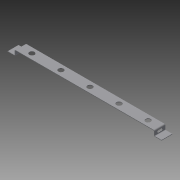
# Autodesk Inventor part: LEDStripOrigami
Saved by Autodesk Inventor 2016 (Build 200138000, 138)
## iProperties
Created: 2015-05-11
Part Number: LEDStripOrigami
Material: Generic
Document SubType Name: Sheet Metal
Designer: Erin
Density: 1 g/cm^3
Sheet Metal Rule: Default_mm
Appearance: Default
Flat Pattern Width: 1 cm
Flat Pattern Length: 15.0524 cm
Flat Pattern Area: 15.0524 cm^2
Sheet Metal Width: 10.000 mm
Sheet Metal Length: 150.524 mm
Sheet Metal Area: 1505.239 mm^2
Author: Erin
Autodesk Inventor part; units mm, degrees
ref_plane "YZ Plane" through (0, 0, 0) normal (1, 0, 0) x (0, 1, 0)
ref_plane "XZ Plane" through (0, 0, 0) normal (0, 1, 0) x (-1, 0, 0)
ref_plane "XY Plane" through (0, 0, 0) normal (0, 0, 1) x (1, 0, 0)
sketch "Sketch1" plane through (0, 0, 0) normal (0, 0, 1) x (1, 0, 0)
  line L0 (-65, 5) -> (65, 5)
  line L1 (65, 5) -> (65, -5)
  line L2 (65, -5) -> (-65, -5)
  line L3 (-65, -5) -> (-65, 5)
  circle A0 centre (0, 0) radius 2.4
  circle A1 centre (-54, 0) radius 2.4
  circle A2 centre (-27, 0) radius 2.4
  circle A3 centre (27, 0) radius 2.4
  circle A4 centre (54, 0) radius 2.4
  line L4 (-65, 0) -> (65, 0) construction
  point P0 (0, 5)
  dimension "d0" = 130
  dimension "d1" = 10
  dimension "d2" = 4.8
  dimension "d3" = 4.8
  dimension "d4" = 4.8
  dimension "d5" = 4.8
  dimension "d6" = 4.8
  dimension "d9" = 27
  dimension "d10" = 27
  dimension "d11" = 27
  dimension "d12" = 27
  measures "d0" distance of L1.end L2.end
  measures "d1" distance of L0.end L1.end
  measures "d2" diameter of A0
  measures "d3" diameter of A1
  measures "d4" diameter of A2
  measures "d5" diameter of A3
  measures "d6" diameter of A4
  measures "d9" distance of A2.centre A0.centre
  measures "d10" distance of A3.centre A0.centre
  measures "d11" distance of A1.centre A2.centre
  measures "d12" distance of A4.centre A3.centre
extrude "Plate1" add sketch "Sketch1" along normal blind 0.5
sketch "Sketch2" plane through (64.5, -5, 0.5) normal (1, 0, 0) x (0, 1, 0)
  line L0 (10, 0) -> (0, 0)
  line L1 (0, 0) -> (0, -5)
  line L2 (0, -5) -> (10, -5)
  line L3 (10, -5) -> (10, 0)
  constraints: 6 end point, 1 horizontal, 1 perpendicular, 1 vertical
edge flange "Flange1" height 5 angle 90 thickness 0.5 bend radius 0.5 thickness toward (1, 0, 0) relief tear relief width 0.5 relief depth 0.25 corner gap 0.5 corner form 0 edges at (65, 0, 0) (-65, 0, 0) wall of the first edge with corners at (64.5, 5, 0.5) (64.5, -5, 0.5) (64.5, -5, -4.5) (64.5, 5, -4.5)
bend "Bend1"
corner "Corner1"
sketch "Sketch3" plane through (64.5, 5, -4) normal (0, 0, -1) x (-1, 0, 0)
  line L0 (0, -10) -> (0, 0)
  line L1 (0, 0) -> (-7, 0)
  line L2 (-7, 0) -> (-7, -10)
  line L3 (-7, -10) -> (0, -10)
  constraints: 6 end point, 1 horizontal, 1 perpendicular, 1 vertical
edge flange "Flange2" height 7 angle 90 thickness 0.5 bend radius 0.5 thickness toward (0, 0, -1) relief tear relief width 0.5 relief depth 0.25 corner gap 0.5 corner form 0 edges at (65, 0, -4.5) (-65, 0, -4.5) wall of the first edge with corners at (64.5, -5, -4) (64.5, 5, -4) (71.5, 5, -4) (71.5, -5, -4)
bend "Bend2"
corner "Corner2"
sketch "Sketch4" plane through (-65, -5, -0.5) normal (-1, 0, 0) x (0, 0, 1)
  line L0 (-3, 10) -> (-3, 0) projected
  line L1 (0, 0) -> (0, 10) projected
  line L2 (-3, 10) -> (0, 10) projected
  line L3 (-1.5, 3.5) -> (-1.5, 6.5) construction
  line L4 (-2.5, 3.5) -> (-2.5, 6.5)
  line L5 (-0.5, 6.5) -> (-0.5, 3.5)
  arc A0 (-2.5, 3.5) -> (-0.5, 3.5) centre (-1.5, 3.5) ccw
  arc A1 (-0.5, 6.5) -> (-2.5, 6.5) centre (-1.5, 6.5) ccw
  point P0 (0.5, 5)
  point P1 (-1.5, 5)
  point P2 (-0.5, 5)
  point P3 (0, 5)
  point P4 (-1.5, 7.5)
  point P5 (-1.5, 10)
  dimension "d34" = 2
  dimension "d35" = 5
  constraints: 8 end point, 5 point on circle, 4 midpoint, 4 tangent, 2 centre point, 2 parallel, 1 horizontal alignment, 1 vertical alignment
  measures "d34" distance between parallel lines of L4 L5
extrude "Cut1" cut sketch "Sketch4" against normal blind 0.5
mirror "Mirror1" about plane through (0, 0, 0) normal (1, 0, 0) of "Cut1"
equation "\"d36\" = Thickness"
equation "\"d14\" = BendReliefWidth"
equation "\"d15\" = BendReliefDepth"
equation "\"d16\" = MinimumRemnant"
equation "\"d17\" = BendRadius"
equation "\"d20\" = BendRadius"
equation "\"d21\" = CornerReliefSize"
equation "\"d22\" = GapSize"
equation "\"d23\" = JacobiRadiusSize"
equation "\"d24\" = BendReliefWidth"
equation "\"d25\" = BendReliefDepth"
equation "\"d26\" = MinimumRemnant"
equation "\"d27\" = BendRadius"
equation "\"d30\" = BendRadius"
equation "\"d31\" = CornerReliefSize"
equation "\"d32\" = GapSize"
equation "\"d33\" = JacobiRadiusSize"
equation "\"BendRadius\" = Thickness"
equation "\"BendReliefWidth\" = Thickness"
equation "\"BendReliefDepth\" = 0.5 * Thickness"
equation "\"CornerReliefSize\" = 4 * Thickness"
equation "\"MinimumRemnant\" = 2 * Thickness"
equation "\"TransitionRadius\" = BendRadius"
equation "\"JacobiRadiusSize\" = BendRadius"
equation "\"GapSize\" = Thickness"
equation "\"kerf\" = 0.2"
equation "\"d13\" = BendRadius"
equation "\"Thickness\" = 0.5"
body "Solid1"
